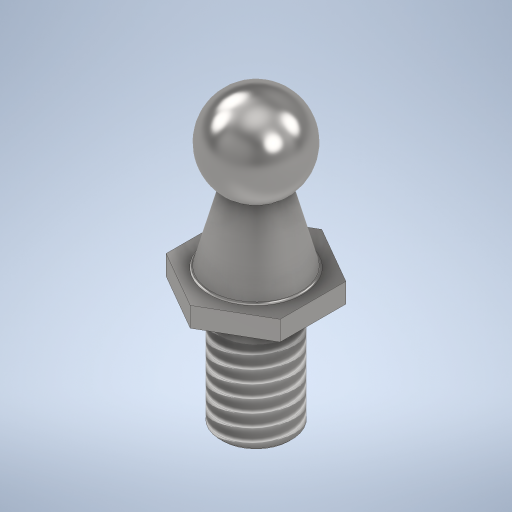
# Autodesk Inventor part: Gas Strut Ball Stud
Saved by Autodesk Inventor 2024 (Build 280153000, 153)
## iProperties
Created: 2024-11-25
Part Number: Gas Strut Ball Stud
Material: Stainless Steel
Document SubType Name: Modeling
Designer: Ishaan
Density: 8 g/cm^3
Appearance: Semi-Polished
Author: Ishaan
Autodesk Inventor part; units mm, degrees
ref_plane "YZ Plane" through (0, 0, 0) normal (1, 0, 0) x (0, 1, 0)
ref_plane "XZ Plane" through (0, 0, 0) normal (0, 1, 0) x (-1, 0, 0)
ref_plane "XY Plane" through (0, 0, 0) normal (0, 0, 1) x (1, 0, 0)
sketch "Sketch1" plane through (0, 0, 0) normal (0, 0, 1) x (1, 0, 0)
  circle A0 centre (0, 0) radius 5
  line L0 (3.9688, -27) -> (-3.9687, -27)
  line L1 (-3.9687, -27) -> (-3.9687, 0)
  line L2 (-3.9687, 0) -> (3.9687, 0)
  line L3 (3.9687, 0) -> (3.9688, -27)
  line L4 (3.9688, -27) -> (-3.9687, 0) construction
  line L5 (-3.9687, -27) -> (3.9687, 0) construction
  line L6 (10, -14.3) -> (-10, -14.3)
  line L7 (-10, -14.3) -> (-10, -12.1)
  line L8 (-10, -12.1) -> (10, -12.1)
  line L9 (10, -12.1) -> (10, -14.3)
  line L10 (10, -14.3) -> (-10, -12.1) construction
  line L11 (-10, -14.3) -> (10, -12.1) construction
  line L12 (-5.0436, -12.1) -> (-2.8939, -4.0774)
  line L13 (2.8939, -4.0774) -> (5.0436, -12.1)
  line L14 (-5.0436, -12.1) -> (5.0436, -12.1) construction
  line L15 (0, 5) -> (0, -27)
  point P0 (0, -13.5)
  point P1 (0, -13.2)
  point P2 (-3.9688, -8.0887)
  point P3 (0, -12.1)
  point P4 (-3.9687, -14.3)
  dimension "d0" = 10
  dimension "d1" = 7.9375
  dimension "d2" = 32
  dimension "d3" = 20
  dimension "d4" = 12.7
  dimension "d5" = 30
  dimension "d6" = 2.2
  constraints: 32 end point, 9 midpoint, 4 parallel, 3 point on circle, 3 point on line, 2 coincident, 2 horizontal, 2 perpendicular, 1 centre point, 1 collinear, 1 equal length, 1 vertical, 1 vertical alignment
  measures "d0" diameter of A0
  measures "d1" distance between parallel lines of L3 L1
  measures "d3" distance of L6.start L6.end
  measures "d4" distance between parallel lines of L0 L6
  measures "d5" angle of L13 L12
  measures "d6" distance between parallel lines of L8 L6
revolve "Revolution1" add sketch "Sketch1" angle 360 about axis through (0, 5, 0) along (0, -1, 0) contours L15 L2 L1 A0 | L1 L2 L15 A0 | A0 L15 L8 L1 L12 | L1 L8 L12 | L8 L15 L6 L1 | L1 L6 L7 L8 | L6 L15 L0 L1
sketch "Sketch2" plane through (0, -14.3, 0) normal (0, -1, 0) x (1, 0, 0)
  circle A0 centre (0, 0) radius 2.8939 projected
  line L0 (-6.35, 3.6662) -> (0, 7.3323)
  line L1 (0, 7.3323) -> (6.35, 3.6662)
  line L2 (6.35, 3.6662) -> (6.35, -3.6662)
  line L3 (6.35, -3.6662) -> (0, -7.3323)
  line L4 (0, -7.3323) -> (-6.35, -3.6662)
  line L5 (-6.35, -3.6662) -> (-6.35, 3.6662)
  circle A1 centre (0, 0) radius 3.9687 projected
  circle A2 centre (0, 0) radius 10 projected
  point P0 (0, 0)
  dimension "d8" = 12.7
  constraints: 12 end point, 1 coincident, 1 vertical, 13 other
  measures "d8" distance between parallel lines of L2 L5
extrude "Extrusion1" cut sketch "Sketch2" against normal through all contours A2
chamfer "Chamfer1" distance 0.25 angle 45 1 edges at (3.9688, -27, 0)
fillet "Fillet1" radius 0.25 1 edges at (3.9688, -14.3, 0)
fillet "Fillet2" radius 0.25 1 edges at (5.0436, -12.1, 0)
thread "Thread1" size "5/16-18 UNC" class "2A" standard "ANSI Unified Screw Threads" length 10
body "Solid1"
